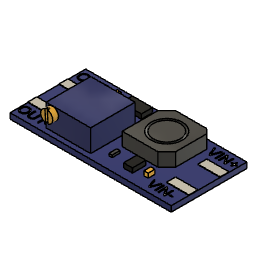
Modulo Step UP v6 (Autodesk Fusion 360 design; units mm, degrees)
Autodesk Fusion 360 part; units mm, degrees
note: some values were not read from the file. Chosen so that the rebuilt part matches the saved one: which bodies a step acts on; the layout of a text. Set by a fixed rule: which sketch regions a step uses.
sketch "Boceto1" plane through (0, 0, 0) normal (0, 1, 0) x (1, 0, 0)
  line L0 (0, 0) -> (36.2, 0)
  line L1 (36.2, 0) -> (36.2, -17)
  line L2 (36.2, -17) -> (0, -17)
  line L3 (0, -17) -> (0, 0)
  dimension "d1" = 36.2
  dimension "d2" = 17
  constraint horizontal L0
  constraint vertical L1
  constraint horizontal L2
  constraint vertical L3
  constraint coincident L0.start L3.end
  measures "d1" distance of L0.start L0.end
  measures "d2" distance of L0.start L2.end
extrude "Extruir1" add sketch "Boceto1" along normal blind 1.25 makes body 1
sketch "Boceto2" plane through (0, 1.25, 0) normal (0, 1, 0) x (-1, 0, 0)
  line L0 (0, 17) -> (-36.2, 17)
  line L1 (-36.2, 17) -> (-36.2, 0)
  line L2 (-36.2, 0) -> (0, 0)
  line L3 (0, 0) -> (0, 17)
  line L4 (0, 0) -> (0, 4)
  line L5 (0, 4) -> (-36.2, 4)
  line L6 (0, 17) -> (0, 13)
  line L7 (0, 13) -> (-36.2, 13)
  line L8 (0, 4) -> (0, 6)
  line L9 (0, 13) -> (0, 11)
  line L10 (-36.2, 13) -> (-36.2, 11)
  line L11 (-36.2, 4) -> (-36.2, 6)
  line L12 (-36.2, 6) -> (-31.2, 6)
  line L13 (-31.2, 6) -> (-31.2, 4)
  line L14 (0, 6) -> (-5, 6)
  line L15 (-5, 6) -> (-5, 4)
  line L16 (0, 11) -> (-5, 11)
  line L17 (-5, 11) -> (-5, 13)
  line L18 (-36.2, 11) -> (-31.2, 11)
  line L19 (-31.2, 11) -> (-31.2, 13)
  dimension "d5" = 4
  dimension "d6" = 4
  dimension "d7" = 2
  dimension "d8" = 5
  dimension "d9" = 5
  dimension "d10" = 5
  constraint coincident L2.end L3.start
  constraint perpendicular L2 L4
  constraint coincident L1 L5.end
  constraint perpendicular L1 L5
  constraint coincident L0.start L3.end
  constraint perpendicular L0 L6
  constraint coincident L1 L7.end
  constraint perpendicular L1 L7
  constraint coincident L3 L8.end
  constraint coincident L3 L9.end
  constraint perpendicular L7 L9
  constraint coincident L1 L10.end
  constraint coincident L1 L11.end
  constraint perpendicular L11 L12
  constraint coincident L5 L13.end
  constraint perpendicular L5 L13
  constraint perpendicular L8 L14
  constraint coincident L5 L15.end
  constraint perpendicular L5 L15
  constraint perpendicular L9 L16
  constraint coincident L7 L17.end
  constraint perpendicular L7 L17
  constraint perpendicular L10 L18
  constraint coincident L7 L19.end
  constraint perpendicular L7 L19
  measures "d5" distance of L2.end L4.end
  measures "d6" distance of L0.start L6.end
  measures "d7" distance of L4.end L8.end
  measures "d8" distance of L11.end L12.end
  measures "d9" distance of L8.end L14.end
  measures "d10" distance of L10.end L18.end
extrude "Extruir2" add sketch "Boceto2" along normal blind 0.1 separate body contours L3 L7 L9 L16 L17 | L1 L7 L10 L18 L19 | L3 L5 L8 L14 L15 | L1 L5 L11 L12 L13 makes body 2 at (32.8667, 1.25, 5.3333) makes body 3 at (3.3333, 1.25, 12.3333) makes body 4 at (3.3333, 1.25, 5.3333) makes body 5 at (32.8667, 1.25, 11.6667)
sketch "Boceto3" plane through (0, 1.25, 0) normal (0, 1, 0) x (-1, 0, 0)
  line L0 (0, 17) -> (-36.2, 17)
  line L1 (-36.2, 17) -> (-36.2, 0)
  line L2 (-36.2, 0) -> (0, 0)
  line L3 (0, 0) -> (0, 17)
  line L4 (0, 17) -> (-7, 17)
  line L5 (-7, 17) -> (-7, 6.9)
  line L6 (-7, 6.9) -> (-17, 6.9)
  line L7 (-17, 6.9) -> (-17, 16.9)
  line L8 (-17, 16.9) -> (-7, 16.9)
  dimension "d15" = 7
  dimension "d16" = 10.1
  dimension "d17" = 10
  dimension "d18" = 10
  dimension "d19" = 10
  constraint coincident L0.start L3.end
  constraint perpendicular L3 L4
  constraint perpendicular L0 L5
  constraint perpendicular L5 L6
  constraint perpendicular L6 L7
  constraint perpendicular L7 L8
  measures "d15" distance of L0.start L4.end
  measures "d16" distance of L4.end L5.end
  measures "d17" distance of L5.end L6.end
  measures "d18" distance of L6.end L7.end
  measures "d19" distance of L7.end L8.end
extrude "Extruir3" add sketch "Boceto3" along normal blind 5 separate body contours L5 L6 L7 L8 makes body 6
sketch "Boceto4" plane through (0, 0, 16.9) normal (0, 0, 1) x (1, 0, 0)
  line L0 (7, 1.25) -> (17, 1.25)
  line L1 (17, 1.25) -> (17, 6.25)
  line L2 (17, 6.25) -> (7, 6.25)
  line L3 (7, 6.25) -> (7, 1.25)
  line L4 (7, 1.25) -> (7, 3.25)
  line L5 (7, 3.25) -> (11, 3.25)
  line L6 (7, 6.25) -> (9, 6.25) construction
  circle A0 centre (8.4142, 4.8358) radius 1.3579
  dimension "d22" = 2
  dimension "d23" = 2
  constraint coincident L0.start L3.end
  constraint perpendicular L0 L4
  constraint perpendicular L4 L5
  constraint horizontal L6
  constraint coincident L2.end L3.start
  measures "d22" distance of L0.start L4.end
  measures "d23" distance of L2.end A0.centre
extrude "Extruir4" add sketch "Boceto4" along normal blind 2 separate body contours A0 makes body 7
sketch "Boceto5" plane through (0, 0, 18.9) normal (0, 0, 1) x (1, 0, 0)
  circle A0 centre (8.4142, 4.8358) radius 1.3579
  line L0 (8.4759, 3.4793) -> (8.3202, 6.1905)
  line L1 (8.0396, 6.141) -> (8.2088, 3.1948)
  line L2 (8.2088, 3.1948) -> (8.7375, 3.2251)
  line L3 (8.7375, 3.2251) -> (8.5676, 6.185)
  constraint coincident A0 L0.start
  constraint coincident A0 L0.end
  constraint coincident A0 L1.start
  constraint parallel L0 L1
  constraint perpendicular L0 L2
  constraint coincident A0 L3.end
  constraint perpendicular L2 L3
extrude "Extruir5" cut sketch "Boceto5" against normal blind 1.2 contours A0 L0 L3 | A0 L0 L1 bodies 7
sketch "Boceto6" plane through (0, 1.25, 0) normal (0, 1, 0) x (-1, 0, 0)
  line L0 (0, 17) -> (-36.2, 17)
  line L1 (-36.2, 17) -> (-36.2, 0)
  line L2 (-36.2, 0) -> (0, 0)
  line L3 (0, 0) -> (0, 17)
  line L4 (-36.2, 0) -> (-29.2, 0)
  line L5 (-29.2, 0) -> (-29.2, 1)
  line L6 (-29.2, 1) -> (-19.2, 1)
  line L7 (-19.2, 1) -> (-19.2, 11)
  line L8 (-19.2, 11) -> (-29.2, 11)
  line L9 (-29.2, 11) -> (-29.2, 1)
  dimension "d29" = 7
  dimension "d30" = 1
  dimension "d31" = 10
  dimension "d32" = 10
  constraint coincident L1.end L2.start
  constraint perpendicular L1 L4
  constraint perpendicular L4 L5
  constraint horizontal L6
  constraint vertical L7
  constraint horizontal L8
  constraint vertical L9
  measures "d29" distance of L1.end L4.end
  measures "d30" distance of L4.end L5.end
  measures "d31" distance of L5.end L6.end
  measures "d32" distance of L5.end L8.end
extrude "Extruir6" add sketch "Boceto6" along normal blind 3 separate body contours L6 L7 L8 L9 makes body 8
sketch "Boceto7" plane through (0, 4.25, 0) normal (0, 1, 0) x (-1, 0, 0)
  line L0 (-29.2, 11) -> (-29.2, 1)
  line L1 (-29.2, 1) -> (-19.2, 1)
  line L2 (-19.2, 1) -> (-19.2, 11)
  line L3 (-19.2, 11) -> (-29.2, 11)
  line L4 (-19.2, 1) -> (-29.2, 11)
  circle A0 centre (-24.2, 6) radius 3
  circle A1 centre (-24.2, 6) radius 3.5
  dimension "d35" = 6
  dimension "d36" = 7
  constraint coincident L1.end L2.start
  constraint coincident L0.start L3.end
  constraint midpoint L4 A0.centre
  constraint concentric A0 A1
  measures "d35" diameter of A0
  measures "d36" diameter of A1
extrude "Extruir7" cut sketch "Boceto7" against normal blind 3 contours L4 A0 A1 | L4 A0 A1 bodies 8 makes body 9 at (20.7174, 3.25, 6.3485)
sketch "Boceto8" plane through (0, 4.25, 0) normal (0, 1, 0) x (-1, 0, 0)
  line L0 (-29.2, 11) -> (-29.2, 1)
  line L1 (-29.2, 1) -> (-19.2, 1)
  line L2 (-19.2, 1) -> (-19.2, 11)
  line L3 (-19.2, 11) -> (-29.2, 11)
  circle A0 centre (-24.2, 6) radius 3.5
  line L4 (-19.2, 1) -> (-19.2, 3)
  line L5 (-19.2, 1) -> (-21.2, 1)
  line L6 (-19.2, 3) -> (-21.2, 1)
  line L7 (-29.2, 11) -> (-27.2, 11)
  line L8 (-29.2, 11) -> (-29.2, 9)
  line L9 (-29.2, 9) -> (-27.2, 11)
  line L10 (-29.2, 1) -> (-29.2, 2)
  line L11 (-29.2, 1) -> (-28.2, 1)
  line L12 (-29.2, 2) -> (-28.2, 1)
  dimension "d39" = 2
  dimension "d40" = 2
  dimension "d41" = 2
  dimension "d42" = 2
  dimension "d43" = 1
  dimension "d44" = 1
  constraint coincident L1.end L2.start
  constraint perpendicular L1 L4
  constraint perpendicular L2 L5
  constraint coincident L0.start L3.end
  constraint perpendicular L0 L7
  constraint perpendicular L7 L8
  constraint coincident L0.end L1.start
  constraint perpendicular L1 L10
  constraint perpendicular L0 L11
  measures "d39" distance of L1.end L4.end
  measures "d40" distance of L1.end L5.end
  measures "d41" distance of L0.start L7.end
  measures "d42" distance of L0.start L8.end
  measures "d43" distance of L0.end L10.end
  measures "d44" distance of L0.end L11.end
extrude "Extruir8" cut sketch "Boceto8" against normal blind 3 contours L0 L3 L7 L8 L9 | L0 L1 L10 L11 L12 | L1 L2 L4 L5 L6 bodies 9
sketch "Boceto9" plane through (0, 1.25, 0) normal (0, 1, 0) x (-1, 0, 0)
  line L0 (0, 17) -> (-36.2, 17)
  line L1 (-36.2, 17) -> (-36.2, 0)
  line L2 (-36.2, 0) -> (0, 0)
  line L3 (0, 0) -> (0, 17)
  line L4 (-0.4042, 3.5) -> (-8.5, 3.5) construction
  line L5 (-8.5, 3.5) -> (-8.5, 0.8493) construction
  line L6 (-8.5, 0.8493) -> (-0.4042, 0.8493) construction
  line L7 (-0.4042, 0.8493) -> (-0.4042, 3.5) construction
  line L8 (-0.1737, 16.5) -> (-8.2695, 16.5) construction
  line L9 (-8.2695, 16.5) -> (-8.2695, 13.8493) construction
  line L10 (-8.2695, 13.8493) -> (-0.1737, 13.8493) construction
  line L11 (-0.1737, 13.8493) -> (-0.1737, 16.5) construction
  line L12 (-29.1737, 16.5) -> (-37.2695, 16.5) construction
  line L13 (-37.2695, 16.5) -> (-37.2695, 13.8493) construction
  line L14 (-37.2695, 13.8493) -> (-29.1737, 13.8493) construction
  line L15 (-29.1737, 13.8493) -> (-29.1737, 16.5) construction
  line L16 (-29.7494, 3.5) -> (-37.8452, 3.5) construction
  line L17 (-37.8452, 3.5) -> (-37.8452, 0.8493) construction
  line L18 (-37.8452, 0.8493) -> (-29.7494, 0.8493) construction
  line L19 (-29.7494, 0.8493) -> (-29.7494, 3.5) construction
  dimension "d47" = 2
  dimension "d48" = 2
  dimension "d49" = 2
  dimension "d50" = 2
  text T0 "OUT+" font "Arial" height 2 align left top in box 8.0958 x 2.6507 at (-0.4042, 3.5) x (-1, 0) y (0, -1) spacing 1
  text T1 "OUT-\n" font "Arial" height 2 align left top in box 8.0958 x 2.6507 at (-0.1737, 16.5) x (-1, 0) y (0, -1) spacing 1 kerned
  text T2 "VIN-\n" font "Arial" height 2 align left top in box 8.0958 x 2.6507 at (-29.1737, 16.5) x (-1, 0) y (0, -1) spacing 1
  text T3 "VIN+\n\n" font "Arial" height 2 align left top in box 8.0958 x 2.6507 at (-29.7494, 3.5) x (-1, 0) y (0, -1) spacing 1
extrude "Extruir9" add sketch "Boceto9" along normal blind 0.01 separate body text T0 T1 T2 T3 makes body 10 at (32.0377, 1.25, 2.1826) makes body 11 at (34.0809, 1.25, 2.0394) makes body 12 at (31.462, 1.25, 15.1826) makes body 13 at (33.5052, 1.25, 15.0394) makes body 14 at (3.9163, 1.25, 14.6192) makes body 15 at (5.1305, 1.25, 15.2613) makes body 16 at (4.1468, 1.25, 1.6192) makes body 17 at (5.361, 1.25, 2.2613) makes body 18 at (7.0213, 1.25, 2.3431) makes body 19 at (0.5051, 1.25, 1.7365) makes body 20 at (6.3738, 1.25, 15.1667) makes body 21 at (0.2746, 1.25, 14.7365) makes body 22 at (34.4106, 1.25, 15.1667) makes body 23 at (29.5379, 1.25, 14.3336) makes body 24 at (35.2492, 1.25, 2.3431) makes body 25 at (30.1136, 1.25, 1.3336)
move_body "Desplazar1" bodies 6 7 to x (1, 0, 0) y (0, 1, 0) z (0, 0, 1) at (0, 0, -1)
extrude "Extruir10" cut 2 faces at (9.3422, 4.7098, 17.9) (7.5248, 5.1541, 17.9) along direction (0, 0, -1) blind 0.7 on bodies 7 bodies 7
sketch "Boceto10" plane through (0, 1.25, 0) normal (0, 1, 0) x (-1, 0, 0)
  line L0 (0, 17) -> (-36.2, 17)
  line L1 (-36.2, 17) -> (-36.2, 0)
  line L2 (-36.2, 0) -> (0, 0)
  line L3 (0, 0) -> (0, 17)
  line L4 (-16, 1) -> (-11.5, 1)
  line L5 (-11.5, 1) -> (-11.5, 3.5)
  line L6 (-11.5, 3.5) -> (-16, 3.5)
  line L7 (-16, 3.5) -> (-16, 1)
  line L8 (-9.5, 1.5) -> (-8.5, 1.5)
  line L9 (-8.5, 1.5) -> (-8.5, 3)
  line L10 (-8.5, 3) -> (-9.5, 3)
  line L11 (-9.5, 3) -> (-9.5, 1.5)
  constraint horizontal L4
  constraint vertical L5
  constraint horizontal L6
  constraint vertical L7
  constraint horizontal L8
  constraint vertical L9
  constraint horizontal L10
  constraint vertical L11
extrude "Extruir11" add sketch "Boceto10" along normal blind 1 separate body contours L4 L5 L6 L7 | L8 L9 L10 L11 makes body 26 at (14.5, 1.25, 2.6667) makes body 27 at (9.1667, 1.25, 2.5)
sketch "Boceto11" plane through (0, 1.25, 0) normal (0, 1, 0) x (-1, 0, 0)
  line L0 (0, 17) -> (-36.2, 17)
  line L1 (-36.2, 17) -> (-36.2, 0)
  line L2 (-36.2, 0) -> (0, 0)
  line L3 (0, 0) -> (0, 17)
  line L4 (-23.5, 12) -> (-25.5, 12)
  line L5 (-25.5, 12) -> (-25.5, 15)
  line L6 (-25.5, 15) -> (-23.5, 15)
  line L7 (-23.5, 15) -> (-23.5, 12)
  line L8 (-19.5, 12.5) -> (-20.2102, 12.5)
  line L9 (-20.2102, 12.5) -> (-20.2102, 14.2658)
  line L10 (-20.2102, 14.2658) -> (-19.5, 14.2658)
  line L11 (-19.5, 14.2658) -> (-19.5, 12.5)
  line L12 (-27.3226, 12.7396) -> (-28.2728, 12.7396)
  line L13 (-28.2728, 12.7396) -> (-28.2728, 14.237)
  line L14 (-28.2728, 14.237) -> (-27.3226, 14.237)
  line L15 (-27.3226, 14.237) -> (-27.3226, 12.7396)
  constraint horizontal L4
  constraint vertical L5
  constraint horizontal L6
  constraint vertical L7
  constraint horizontal L8
  constraint vertical L9
  constraint horizontal L10
  constraint vertical L11
  constraint horizontal L12
  constraint vertical L13
  constraint horizontal L14
  constraint vertical L15
extrude "Extruir12" add sketch "Boceto11" along normal blind 1 separate body contours L4 L5 L6 L7 | L12 L13 L14 L15 makes body 28 at (28.2728, 1.5833, 13.2388) makes body 29 at (24.1667, 1.25, 13)
extrude "Extruir13" add sketch "Boceto11" along normal blind 0.5 separate body contours L8 L9 L10 L11 makes body 30
